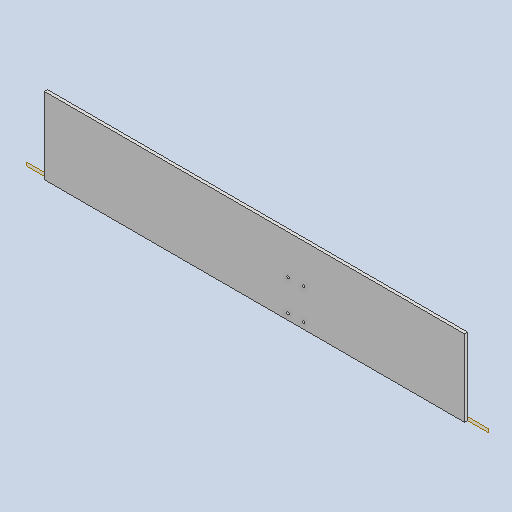
# Autodesk Inventor part: top_plate
Saved by Autodesk Inventor 2022 (Build 260153000, 153)
## iProperties
Created: 2021-07-14
Part Number: top_plate
Material: Generic
Document SubType Name: Modeling
Designer: gfellows
Density: 1 g/cm^3
Appearance: Default
Author: gfellows
Autodesk Inventor part; units mm, degrees
ref_plane "YZ Plane" through (0, 0, 0) normal (1, 0, 0) x (0, 1, 0)
ref_plane "XZ Plane" through (0, 0, 0) normal (0, 1, 0) x (-1, 0, 0)
ref_plane "XY Plane" through (0, 0, 0) normal (0, 0, 1) x (1, 0, 0)
ref_plane "Work Plane1" through (-371.7905, 0, 55) normal (0, 0, 1) x (1, 0, 0)
sketch "Sketch1" plane through (-371.7905, 0, 55) normal (0, 0, 1) x (1, 0, 0)
  line L0 (0, 0) -> (430.2, 0)
  line L1 (430.2, 0) -> (430.2, 78.35)
  line L2 (430.2, 78.35) -> (0, 78.35)
  line L3 (0, 78.35) -> (0, 0)
  circle A0 centre (265.5182, 6.225) radius 1.3525 projected
  line L4 (232.7522, 3.429) -> (232.7522, 41.021) projected
  line L5 (271.9952, 3.429) -> (232.7522, 3.429) projected
  line L6 (271.9952, 41.021) -> (271.9952, 3.429) projected
  line L7 (232.7522, 41.021) -> (271.9952, 41.021) projected
  circle A1 centre (265.5182, 6.225) radius 1.3525 projected
  circle A2 centre (249.5182, 6.225) radius 1.3525 projected
  circle A3 centre (265.5182, 38.225) radius 1.3525 projected
  circle A4 centre (249.5182, 38.225) radius 1.3525 projected
  point P0 (371.7905, 0)
  constraints: 8 end point, 2 parallel, 1 horizontal, 1 perpendicular, 2 other
extrude "Extrusion1" add sketch "Sketch1" along normal blind 3.175 contours L3 L2 L1 L0 | L4 L7 L6 L5
body "Solid1"
